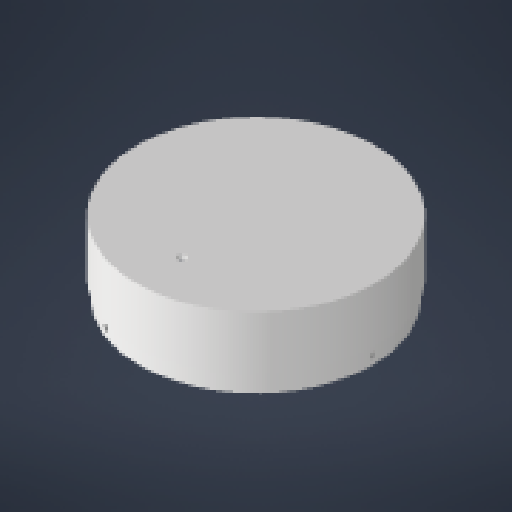
# Autodesk Inventor part: Abdeckung_Gaseinlass_new
Saved by Autodesk Inventor 2027 (Build 310192060, 192F)
## iProperties
Created: 2026-07-15
Part Number: Abdeckung_Gaseinlass_new
Material: Generic
Document SubType Name: Modeling
Designer: kw
Density: 1 g/cm^3
Appearance: Default
Author: kw
Autodesk Inventor part; units mm, degrees
note: some values were not read from the file. Chosen so that the rebuilt part matches the saved one: pattern direction of "Circular Pattern6".
ref_plane "XZ Plane" through (0, 0, 0) normal (0, 1, 0) x (-1, 0, 0)
ref_plane "XY Plane" through (0, 0, 0) normal (0, 0, 1) x (1, 0, 0)
sketch "Sketch1" plane through (0, 0, 0) normal (0, 1, 0) x (-1, 0, 0)
  circle A0 centre (0, 0) radius 47
  circle A1 centre (0, 0) radius 43
  dimension "d0" = 94
  dimension "d8" = 4
  constraints: 2 centre point, 1 coincident
  measures "d0" diameter of A0
  measures "d8" radial gap between concentric circles of A0 A1
extrude "Extrusion1" add sketch "Sketch1" along normal blind 7
sketch "Sketch2" plane through (0, 7, 0) normal (0, 1, 0) x (1, 0, 0)
  circle A0 centre (0, 0) radius 43
  circle A1 centre (0, 0) radius 48
  dimension "d38" = 86
  dimension "d39" = 96
  constraints: 2 centre point, 1 coincident
  measures "d38" diameter of A0
  measures "d39" diameter of A1
extrude "Extrusion2" add sketch "Sketch2" along normal blind 20
sketch "Sketch6" plane through (0, 27, 0) normal (0, 1, 0) x (1, 0, 0)
  circle A0 centre (0, 0) radius 48 projected
extrude "Extrusion5" add sketch "Sketch6" along normal blind 2
ref_plane "Work Plane2" through (47, 0, 0) normal (1, 0, 0) x (0, 1, 0)
sketch "Sketch7" plane through (47, 0, 0) normal (1, 0, 0) x (0, 1, 0)
  point P0 (0, 0)
  point P1 (3.5, 0)
hole "Hole1" at (47, 3.5, 0) direction (-1, 0, 0) diameter 2.459 depth 5 thread size "M3x0.5" class "6H" standard "ISO Metric profile"
pattern_circular "Circular Pattern6" count 3 over 220 about axis through (0, 0, 0) along (0, 1, 0) of "Hole1" both ways yes
sketch "Sketch8" plane through (0, 29, 0) normal (0, 1, 0) x (1, 0, 0)
  circle A0 centre (0, -30) radius 1.55
  point P0 (0, 0)
  dimension "d62" = 3.1
  constraints: 1 centre point
  measures "d62" diameter of A0
extrude "Extrusion6" cut sketch "Sketch8" against normal blind 2
body "Solid1"
